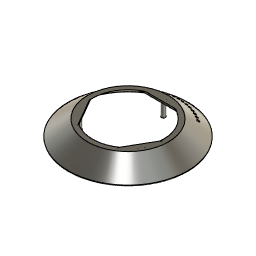
benderbase (Autodesk Fusion 360 design; units mm, degrees)
Autodesk Fusion 360 part; units mm, degrees
note: some values were not read from the file. Set by a fixed rule: which face or edge a step refers to.
sketch "Sketch1" plane through (0, 0, 0) normal (0, 0, 1) x (1, 0, 0)
  circle A0 centre (0, 0) radius 75
  dimension "d1" = 150
  constraint coincident A0.centre origin
  measures "d1" diameter of A0
sketch "Sketch2" plane through (0, 0, 20) normal (0, 0, 1) x (1, 0, 0)
  circle A0 centre (0, 0) radius 50
  dimension "d4" = 100
  constraint coincident A0.centre origin
  measures "d4" diameter of A0
loft "Loft1" add profiles "Sketch2", "Sketch1" section 1 section 2 makes body 1
shell "Shell1" thickness 3.75 removed faces 1 at (-13.5518, -2.484, 20) on bodies 1
delete_face "DeleteFace1" 1 faces at (-20.0266, 12.4245, 3.75) on bodies 1
hole "Hole1" at (0, 61.2217, 11.0226) direction (0, -0.624695, -0.780869) diameter 3 depth 30 tip angle 118 bodies 1
delete_face "DeleteFace3" 1 faces at (0.1037, 61.6093, 9.1116) on bodies 1
sketch "Sketch3" plane through (0, 0, 0) normal (0, 0, 1) x (1, 0, 0)
  circle A0 centre (-0.1874, 62.4997) radius 1.5
  circle A1 centre (-5.6339, 62.2456) radius 1.5
  circle A2 centre (-11.0375, 61.5177) radius 1.5
  circle A3 centre (-16.3571, 60.3216) radius 1.5
  circle A4 centre (-21.5522, 58.6664) radius 1.5
  circle A5 centre (-26.5833, 56.5648) radius 1.5
  circle A6 centre (-31.4121, 54.0327) radius 1.5
  circle A7 centre (-36.0019, 51.0893) radius 1.5
  circle A8 centre (5.2605, 62.2782) radius 1.5
  circle A9 centre (10.6684, 61.5827) radius 1.5
  circle A10 centre (15.9951, 60.4186) radius 1.5
  circle A11 centre (21.2001, 58.7946) radius 1.5
  circle A12 centre (26.2437, 56.7232) radius 1.5
  circle A13 centre (31.0876, 54.22) radius 1.5
  circle A14 centre (35.6949, 51.3043) radius 1.5
  dimension "d10" = 3
  dimension "d11" = 3
  dimension "d12" = 3
  dimension "d13" = 3
  dimension "d14" = 3
  dimension "d15" = 3
  dimension "d16" = 3
  dimension "d17" = 3
  dimension "d18" = 3
  dimension "d19" = 3
  dimension "d20" = 3
  dimension "d21" = 3
  dimension "d22" = 3
  dimension "d23" = 3
  dimension "d24" = 3
  measures "d10" diameter of A0
  measures "d11" diameter of A1
  measures "d12" diameter of A2
  measures "d13" diameter of A3
  measures "d14" diameter of A4
  measures "d15" diameter of A5
  measures "d16" diameter of A6
  measures "d17" diameter of A7
  measures "d18" diameter of A8
  measures "d19" diameter of A9
  measures "d20" diameter of A10
  measures "d21" diameter of A11
  measures "d22" diameter of A12
  measures "d23" diameter of A13
  measures "d24" diameter of A14
extrude "Extrude1" cut sketch "Sketch3" along normal blind 21 bodies 1
fillet "Fillet1" radius 0.5 1 edges at (-69.9246, -27.1212, 0) on bodies 1
fillet "Fillet2" radius 1 1 edges at (-64.3279, 24.9504, 0) on bodies 1
sketch "Sketch4" plane through (0, 0, 0) normal (0, 0, 1) x (1, 0, 0)
  line L0 (-19, 40) -> (19, 40)
  line L1 (19, 40) -> (19, 45)
  line L2 (19, 45) -> (-19, 45)
  line L3 (-19, 45) -> (-19, 40)
  constraint horizontal L0
  constraint vertical L1
  constraint horizontal L2
  constraint vertical L3
extrude "Extrude2" add sketch "Sketch4" along normal blind 20 separate body makes body 2
copy_body "CopyPasteBodies1" bodies 2 makes body 3
move_body "Move1" bodies 3 to x (-0.5, -0.866025, 0) y (0.866025, -0.5, 0) z (0, 0, 1) at (0, 0, 0)
copy_body "CopyPasteBodies2" bodies 2 makes body 4
move_body "Move2" bodies 4 to x (-0.5, 0.866025, 0) y (-0.866025, -0.5, 0) z (0, 0, 1) at (0, 0, 0)
move_face "OffsetFaces1" offset -18 3 faces at (-6.3333, 43.3333, 0) (39.2511, -15.3485, 0) (-40.6944, -16.1818, 0) on bodies 2 3 4
combine "Combine1" operation add target body 3 tool bodies 4 2 1
move_face "OffsetFaces2" offset 4.5 1 faces at (19, 40.6008, 18.7456) on bodies 3
move_face "OffsetFaces3" offset 4.5 1 faces at (-19, 40.6008, 18.7456) on bodies 3
move_face "OffsetFaces4" offset 4.5 1 faces at (-44.6613, -3.8459, 18.7456) on bodies 3
move_face "OffsetFaces5" offset 4.5 1 faces at (-25.6613, -36.7549, 18.7456) on bodies 3
move_face "OffsetFaces6" offset 4.5 1 faces at (25.6613, -36.7549, 18.7456) on bodies 3
move_face "OffsetFaces7" offset 4.5 1 faces at (44.6613, -3.8459, 18.7456) on bodies 3
sketch "Sketch5" plane through (0, 0, 0) normal (0, 0, 1) x (1, 0, 0)
  circle A0 centre (38.1051, -22) radius 2.5
  dimension "d42" = 5
  measures "d42" diameter of A0
sketch "Sketch6" plane through (0, 0, 0) normal (0, 0, 1) x (1, 0, 0)
  circle A0 centre (0, 44) radius 2.5
  dimension "d43" = 5
  measures "d43" diameter of A0
sketch "Sketch7" plane through (0, 0, 0) normal (0, 0, 1) x (1, 0, 0)
  circle A0 centre (-38.1051, -22) radius 2.5
  dimension "d44" = 5
  measures "d44" diameter of A0
extrude "Extrude3" add sketch "Sketch5" sketch "Sketch6" sketch "Sketch7" along normal blind 20 of sketch 2 of sketch 3 bodies 3
fillet "Fillet3" radius 0.5 3 edges at (-2.3308, 43.096, 0) (-36.1568, -23.5665, 0) (38.4876, -19.5294, 0) on bodies 3
